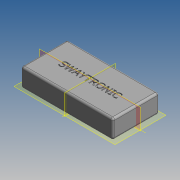
# Autodesk Inventor part: P025_Batterie
Saved by Autodesk Inventor 2021.3 (Build 253353000, 353)
## iProperties
Created: 2021-11-19
Part Number: P025_Batterie
Material: Générique
Document SubType Name: Modeling
Designer: gabri
Density: 1 g/cm^3
Appearance: Par défaut
Author: gabri
Autodesk Inventor part; units mm, degrees
sketch "Sketch2" plane through (0, 0, 0) normal (0, 0, 1) x (1, 0, 0)
  line L0 (46.5, -23.5) -> (-46.5, -23.5)
  line L1 (-46.5, -23.5) -> (-46.5, 23.5)
  line L2 (-46.5, 23.5) -> (46.5, 23.5)
  line L3 (46.5, 23.5) -> (46.5, -23.5)
  line L4 (46.5, -23.5) -> (-46.5, 23.5) construction
  line L5 (-46.5, -23.5) -> (46.5, 23.5) construction
  point P0 (0, 0)
  dimension "d0" = 93
  dimension "d1" = 47
  constraints: 12 end point, 2 midpoint, 2 parallel, 1 horizontal, 1 perpendicular
  measures "d0" distance of L1.end L2.end
  measures "d1" distance of L0.end L1.end
extrude "Extrusion1" add sketch "Sketch2" along normal blind 19
fillet "Fillet1" radius 2 12 edges at (-46.5, -23.5, 9.5) (46.5, -23.5, 9.5) (46.5, 23.5, 9.5) (-46.5, 23.5, 9.5) (0, 23.5, 19) (-46.5, 0, 19) (0, -23.5, 19) (46.5, 0, 19) (0, -23.5, 0) (46.5, 0, 0) (-46.5, 0, 0) (0, 23.5, 0)
sketch "Sketch3" plane through (0, 0, 19) normal (0, 0, 1) x (1, 0, 0)
  line L0 (-29.2409, 3.321) -> (13.3077, 3.321) construction
  line L1 (13.3077, 3.321) -> (13.3077, -3.0237) construction
  line L2 (13.3077, -3.0237) -> (-29.2409, -3.0237) construction
  line L3 (-29.2409, -3.0237) -> (-29.2409, 3.321) construction
  spline S0 degree 2 poles (-26.5805, -3.9513) (-27.3406, -3.9513) (-28.4071, -3.6336) (-28.8779, -3.4067) knots 0 0 0 1 2 2 2
  line L4 (-28.8779, -3.4067) -> (-28.8779, -2.2382)
  line L5 (-28.8779, -2.2382) -> (-28.8098, -2.2382)
  spline S1 degree 2 poles (-28.8098, -2.2382) (-28.3503, -2.6693) (-27.1874, -3.1458) (-26.6485, -3.1458) knots 0 0 0 1 2 2 2
  spline S2 degree 2 poles (-26.6485, -3.1458) (-25.8771, -3.1458) (-25.0886, -2.5048) (-25.0886, -1.9772) knots 0 0 0 1 2 2 2
  spline S3 degree 2 poles (-25.0886, -1.9772) (-25.0886, -1.5575) (-25.5027, -1.0356) (-25.9508, -0.9051) knots 0 0 0 1 2 2 2
  spline S4 degree 2 poles (-25.9508, -0.9051) (-26.2742, -0.8143) (-26.813, -0.6895) (-27.2158, -0.5874) knots 0 0 0 1 2 2 2
  spline S5 degree 2 poles (-27.2158, -0.5874) (-27.5789, -0.491) (-28.1518, -0.2017) (-28.373, 0.0309) knots 0 0 0 1 2 2 2
  spline S6 degree 2 poles (-28.373, 0.0309) (-28.5886, 0.2635) (-28.8268, 0.8874) (-28.8268, 1.2959) knots 0 0 0 1 2 2 2
  spline S7 degree 2 poles (-28.8268, 1.2959) (-28.8268, 2.1468) (-27.4994, 3.2983) (-26.4727, 3.2983) knots 0 0 0 1 2 2 2
  spline S8 degree 2 poles (-26.4727, 3.2983) (-25.8827, 3.2983) (-24.839, 3.0657) (-24.3908, 2.8445) knots 0 0 0 1 2 2 2
  line L6 (-24.3908, 2.8445) -> (-24.3908, 1.7327)
  line L7 (-24.3908, 1.7327) -> (-24.4589, 1.7327)
  spline S9 degree 2 poles (-24.4589, 1.7327) (-24.7936, 2.039) (-25.8374, 2.4928) (-26.4103, 2.4928) knots 0 0 0 1 2 2 2
  spline S10 degree 2 poles (-26.4103, 2.4928) (-27.057, 2.4928) (-27.8568, 1.8858) (-27.8568, 1.3923) knots 0 0 0 1 2 2 2
  spline S11 degree 2 poles (-27.8568, 1.3923) (-27.8568, 0.9498) (-27.386, 0.4223) (-26.9435, 0.3032) knots 0 0 0 1 2 2 2
  spline S12 degree 2 poles (-26.9435, 0.3032) (-26.6485, 0.2237) (-25.792, 0.0195) (-25.5083, -0.0656) knots 0 0 0 1 2 2 2
  spline S13 degree 2 poles (-25.5083, -0.0656) (-24.7879, -0.2868) (-24.1186, -1.1774) (-24.1186, -1.8297) knots 0 0 0 1 2 2 2
  spline S14 degree 2 poles (-24.1186, -1.8297) (-24.1186, -2.2438) (-24.4532, -3.038) (-24.7539, -3.316) knots 0 0 0 1 2 2 2
  spline S15 degree 2 poles (-24.7539, -3.316) (-25.0886, -3.6223) (-25.9395, -3.9513) (-26.5805, -3.9513) knots 0 0 0 1 2 2 2
  line L8 (-15.326, 3.1735) -> (-17.0845, -3.8265)
  line L9 (-17.0845, -3.8265) -> (-18.1283, -3.8265)
  line L10 (-18.1283, -3.8265) -> (-19.5521, 1.9823)
  line L11 (-19.5521, 1.9823) -> (-20.9362, -3.8265)
  line L12 (-20.9362, -3.8265) -> (-21.9686, -3.8265)
  line L13 (-21.9686, -3.8265) -> (-23.7555, 3.1735)
  line L14 (-23.7555, 3.1735) -> (-22.7968, 3.1735)
  line L15 (-22.7968, 3.1735) -> (-21.39, -2.6296)
  line L16 (-21.39, -2.6296) -> (-19.9946, 3.1735)
  line L17 (-19.9946, 3.1735) -> (-19.0472, 3.1735)
  line L18 (-19.0472, 3.1735) -> (-17.6404, -2.6976)
  line L19 (-17.6404, -2.6976) -> (-16.2393, 3.1735)
  line L20 (-16.2393, 3.1735) -> (-15.326, 3.1735)
  line L21 (-15.2466, -3.8265) -> (-12.8868, 3.1735)
  line L22 (-12.8868, 3.1735) -> (-11.7409, 3.1735)
  line L23 (-11.7409, 3.1735) -> (-9.3811, -3.8265)
  line L24 (-9.3811, -3.8265) -> (-10.3625, -3.8265)
  line L25 (-10.3625, -3.8265) -> (-10.9978, -1.8694)
  line L26 (-10.9978, -1.8694) -> (-13.6696, -1.8694)
  line L27 (-13.6696, -1.8694) -> (-14.3049, -3.8265)
  line L28 (-14.3049, -3.8265) -> (-15.2466, -3.8265)
  line L29 (-11.2531, -1.0753) -> (-12.3365, 2.2205)
  line L30 (-12.3365, 2.2205) -> (-13.4143, -1.0753)
  line L31 (-13.4143, -1.0753) -> (-11.2531, -1.0753)
  line L32 (-3.8163, 3.1735) -> (-6.1818, -0.7293)
  line L33 (-6.1818, -0.7293) -> (-6.1818, -3.8265)
  line L34 (-6.1818, -3.8265) -> (-7.1121, -3.8265)
  line L35 (-7.1121, -3.8265) -> (-7.1121, -0.8257)
  line L36 (-7.1121, -0.8257) -> (-9.4776, 3.1735)
  line L37 (-9.4776, 3.1735) -> (-8.4451, 3.1735)
  line L38 (-8.4451, 3.1735) -> (-6.6412, 0.0933)
  line L39 (-6.6412, 0.0933) -> (-4.8033, 3.1735)
  line L40 (-4.8033, 3.1735) -> (-3.8163, 3.1735)
  line L41 (-1.5359, -3.8265) -> (-1.5359, 2.3453)
  line L42 (-1.5359, 2.3453) -> (-3.8844, 2.3453)
  line L43 (-3.8844, 2.3453) -> (-3.8844, 3.1735)
  line L44 (-3.8844, 3.1735) -> (1.7429, 3.1735)
  line L45 (1.7429, 3.1735) -> (1.7429, 2.3453)
  line L46 (1.7429, 2.3453) -> (-0.6056, 2.3453)
  line L47 (-0.6056, 2.3453) -> (-0.6056, -3.8265)
  line L48 (-0.6056, -3.8265) -> (-1.5359, -3.8265)
  line L49 (7.8693, -3.8265) -> (6.661, -3.8265)
  line L50 (6.661, -3.8265) -> (4.4487, -1.0412)
  line L51 (4.4487, -1.0412) -> (3.3823, -1.0412)
  line L52 (3.3823, -1.0412) -> (3.3823, -3.8265)
  line L53 (3.3823, -3.8265) -> (2.4519, -3.8265)
  line L54 (2.4519, -3.8265) -> (2.4519, 3.1735)
  line L55 (2.4519, 3.1735) -> (4.2558, 3.1735)
  spline S16 degree 2 poles (4.2558, 3.1735) (4.8571, 3.1735) (5.6683, 3.043) (6.037, 2.8048) knots 0 0 0 1 2 2 2
  spline S17 degree 2 poles (6.037, 2.8048) (6.4058, 2.5665) (6.8312, 1.8234) (6.8312, 1.2732) knots 0 0 0 1 2 2 2
  spline S18 degree 2 poles (6.8312, 1.2732) (6.8312, 0.5074) (6.0484, -0.5307) (5.379, -0.7803) knots 0 0 0 1 2 2 2
  line L56 (5.379, -0.7803) -> (7.8693, -3.8265)
  spline S19 degree 2 poles (5.8612, 1.1994) (5.8612, 1.5058) (5.6456, 1.9766) (5.4187, 2.1297) knots 0 0 0 1 2 2 2
  spline S20 degree 2 poles (5.4187, 2.1297) (5.2202, 2.2602) (4.6926, 2.368) (4.3069, 2.368) knots 0 0 0 1 2 2 2
  line L57 (4.3069, 2.368) -> (3.3823, 2.368)
  line L58 (3.3823, 2.368) -> (3.3823, -0.2641)
  line L59 (3.3823, -0.2641) -> (4.1991, -0.2641)
  spline S21 degree 2 poles (4.1991, -0.2641) (4.6019, -0.2641) (5.2429, -0.1223) (5.4641, 0.0989) knots 0 0 0 1 2 2 2
  spline S22 degree 2 poles (5.4641, 0.0989) (5.6683, 0.2918) (5.8612, 0.8364) (5.8612, 1.1994) knots 0 0 0 1 2 2 2
  spline S23 degree 2 poles (13.3774, 2.3737) (13.7745, 1.9085) (14.2169, 0.5471) (14.2169, -0.3265) knots 0 0 0 1 2 2 2
  spline S24 degree 2 poles (14.2169, -0.3265) (14.2169, -1.1774) (13.7858, -2.5558) (13.3774, -3.021) knots 0 0 0 1 2 2 2
  spline S25 degree 2 poles (13.3774, -3.021) (12.9463, -3.5088) (11.8061, -3.974) (11.1197, -3.974) knots 0 0 0 1 2 2 2
  spline S26 degree 2 poles (11.1197, -3.974) (10.4106, -3.974) (9.2761, -3.4918) (8.862, -3.021) knots 0 0 0 1 2 2 2
  spline S27 degree 2 poles (8.862, -3.021) (8.4592, -2.5558) (8.0281, -1.1887) (8.0281, -0.3265) knots 0 0 0 1 2 2 2
  spline S28 degree 2 poles (8.0281, -0.3265) (8.0281, 0.5528) (8.4649, 1.8915) (8.8677, 2.3737) knots 0 0 0 1 2 2 2
  spline S29 degree 2 poles (8.8677, 2.3737) (9.2761, 2.8388) (10.4163, 3.321) (11.1197, 3.321) knots 0 0 0 1 2 2 2
  spline S30 degree 2 poles (11.1197, 3.321) (11.8344, 3.321) (12.9803, 2.8218) (13.3774, 2.3737) knots 0 0 0 1 2 2 2
  spline S31 degree 2 poles (13.2469, -0.3265) (13.2469, 0.3656) (12.9463, 1.4377) (12.674, 1.7894) knots 0 0 0 1 2 2 2
  spline S32 degree 2 poles (12.674, 1.7894) (12.396, 2.1524) (11.6132, 2.5155) (11.1254, 2.5155) knots 0 0 0 1 2 2 2
  spline S33 degree 2 poles (11.1254, 2.5155) (10.6205, 2.5155) (9.8604, 2.1638) (9.5711, 1.7894) knots 0 0 0 1 2 2 2
  spline S34 degree 2 poles (9.5711, 1.7894) (9.2931, 1.432) (8.9981, 0.3542) (8.9981, -0.3265) knots 0 0 0 1 2 2 2
  spline S35 degree 2 poles (8.9981, -0.3265) (8.9981, -1.7049) (10.1553, -3.1685) (11.1254, -3.1685) knots 0 0 0 1 2 2 2
  spline S36 degree 2 poles (11.1254, -3.1685) (12.0954, -3.1685) (13.2469, -1.7049) (13.2469, -0.3265) knots 0 0 0 1 2 2 2
  line L60 (20.2469, -3.8265) -> (19.2032, -3.8265)
  line L61 (19.2032, -3.8265) -> (16.1059, 2.2092)
  line L62 (16.1059, 2.2092) -> (16.1059, -3.8265)
  line L63 (16.1059, -3.8265) -> (15.238, -3.8265)
  line L64 (15.238, -3.8265) -> (15.238, 3.1735)
  line L65 (15.238, 3.1735) -> (16.5597, 3.1735)
  line L66 (16.5597, 3.1735) -> (19.379, -2.3686)
  line L67 (19.379, -2.3686) -> (19.379, 3.1735)
  line L68 (19.379, 3.1735) -> (20.2469, 3.1735)
  line L69 (20.2469, 3.1735) -> (20.2469, -3.8265)
  line L70 (24.1043, -3.8265) -> (21.3928, -3.8265)
  line L71 (21.3928, -3.8265) -> (21.3928, -3.1117)
  line L72 (21.3928, -3.1117) -> (22.2834, -3.1117)
  line L73 (22.2834, -3.1117) -> (22.2834, 2.4588)
  line L74 (22.2834, 2.4588) -> (21.3928, 2.4588)
  line L75 (21.3928, 2.4588) -> (21.3928, 3.1735)
  line L76 (21.3928, 3.1735) -> (24.1043, 3.1735)
  line L77 (24.1043, 3.1735) -> (24.1043, 2.4588)
  line L78 (24.1043, 2.4588) -> (23.2137, 2.4588)
  line L79 (23.2137, 2.4588) -> (23.2137, -3.1117)
  line L80 (23.2137, -3.1117) -> (24.1043, -3.1117)
  line L81 (24.1043, -3.1117) -> (24.1043, -3.8265)
  spline S37 degree 2 poles (27.99, -3.9513) (27.3093, -3.9513) (26.1578, -3.4918) (25.738, -3.0323) knots 0 0 0 1 2 2 2
  spline S38 degree 2 poles (25.738, -3.0323) (25.3182, -2.5785) (24.8588, -1.2171) (24.8588, -0.3322) knots 0 0 0 1 2 2 2
  spline S39 degree 2 poles (24.8588, -0.3322) (24.8588, 0.5471) (25.3069, 1.8518) (25.7323, 2.334) knots 0 0 0 1 2 2 2
  spline S40 degree 2 poles (25.7323, 2.334) (26.1521, 2.8048) (27.298, 3.2983) (28.007, 3.2983) knots 0 0 0 1 2 2 2
  spline S41 degree 2 poles (28.007, 3.2983) (28.3588, 3.2983) (28.9771, 3.1962) (29.238, 3.1168) knots 0 0 0 1 2 2 2
  spline S42 degree 2 poles (29.238, 3.1168) (29.4649, 3.043) (29.9357, 2.8331) (30.1683, 2.7083) knots 0 0 0 1 2 2 2
  line L82 (30.1683, 2.7083) -> (30.1683, 1.5852)
  line L83 (30.1683, 1.5852) -> (30.0946, 1.5852)
  spline S43 degree 2 poles (30.0946, 1.5852) (29.9698, 1.6986) (29.584, 2.0163) (29.3061, 2.1695) knots 0 0 0 1 2 2 2
  spline S44 degree 2 poles (29.3061, 2.1695) (29.0395, 2.3169) (28.4098, 2.5041) (28.0014, 2.5041) knots 0 0 0 1 2 2 2
  spline S45 degree 2 poles (28.0014, 2.5041) (27.5532, 2.5041) (26.7534, 2.1354) (26.4528, 1.7837) knots 0 0 0 1 2 2 2
  spline S46 degree 2 poles (26.4528, 1.7837) (26.1578, 1.4263) (25.8288, 0.3429) (25.8288, -0.3322) knots 0 0 0 1 2 2 2
  spline S47 degree 2 poles (25.8288, -0.3322) (25.8288, -1.0526) (26.1748, -2.0907) (26.4754, -2.4481) knots 0 0 0 1 2 2 2
  spline S48 degree 2 poles (26.4754, -2.4481) (26.7704, -2.7941) (27.5589, -3.1458) (28.0014, -3.1458) knots 0 0 0 1 2 2 2
  spline S49 degree 2 poles (28.0014, -3.1458) (28.4041, -3.1458) (29.0905, -2.9472) (29.3571, -2.7998) knots 0 0 0 1 2 2 2
  spline S50 degree 2 poles (29.3571, -2.7998) (29.6124, -2.6523) (29.9925, -2.3459) (30.1002, -2.2382) knots 0 0 0 1 2 2 2
  line L84 (30.1002, -2.2382) -> (30.1683, -2.2382)
  line L85 (30.1683, -2.2382) -> (30.1683, -3.35)
  spline S51 degree 2 poles (30.1683, -3.35) (29.9357, -3.4578) (29.5273, -3.6563) (29.238, -3.7471) knots 0 0 0 1 2 2 2
  spline S52 degree 2 poles (29.238, -3.7471) (28.9317, -3.8492) (28.4098, -3.9513) (27.99, -3.9513) knots 0 0 0 1 2 2 2
  point P0 (0, 0)
  constraints: 2 other
emboss "Emboss1" sketch "Sketch3" operation cut depth 1 direction (0, 0, -1)
body "Solid1"
